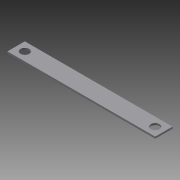
# Autodesk Inventor part: 4barBar
Saved by Autodesk Inventor 2015 SP1 (Build 190203100, 203)
## iProperties
Created: 2015-02-16
Part Number: 4barBar
Material: Generic
Document SubType Name: Modeling
Designer: 55221
Density: 1 g/cm^3
Appearance: Default
Author: 55221
Autodesk Inventor part; units mm, degrees
ref_plane "YZ Plane" through (0, 0, 0) normal (1, 0, 0) x (0, 1, 0)
ref_plane "XZ Plane" through (0, 0, 0) normal (0, 1, 0) x (-1, 0, 0)
ref_plane "XY Plane" through (0, 0, 0) normal (0, 0, 1) x (1, 0, 0)
sketch "Sketch1" plane through (0, 0, 0) normal (0, 1, 0) x (-1, 0, 0)
  line L0 (203.2, 25.4) -> (0, 25.4)
  line L1 (0, 25.4) -> (0, 0)
  line L2 (0, 0) -> (203.2, 0)
  line L3 (203.2, 0) -> (203.2, 25.4)
  constraints: 8 end point, 2 parallel, 1 horizontal, 1 perpendicular
extrude "Extrusion1" add sketch "Sketch1" along normal blind 2.54
sketch "Sketch2" plane through (0, 2.54, 0) normal (0, 1, 0) x (1, 0, 0)
  circle A0 centre (-12.7, -12.7) radius 6.35
  point P0 (0, 0)
  dimension "d2" = 12.7
  constraints: 1 centre point
  measures "d2" diameter of A0
sketch "Sketch3" plane through (-203.2, 0, 0) normal (-1, 0, 0) x (0, 0, 1)
  line L0 (25.4, 0) -> (0, 0) projected
  line L1 (25.4, 0) -> (25.4, 2.54) projected
  line L2 (0, 2.54) -> (25.4, 2.54) projected
  line L3 (0, 0) -> (0, 2.54) projected
extrude "Extrusion2" add sketch "Sketch3" along normal blind 12.7
sketch "Sketch4" plane through (0, 2.54, 0) normal (0, 1, 0) x (1, 0, 0)
  circle A0 centre (-203.2, -12.7) radius 6.35
  point P0 (0, 0)
  dimension "d5" = 12.7
  constraints: 1 centre point
  measures "d5" diameter of A0
extrude "Extrusion3" cut sketch "Sketch4" against normal blind 2.54
extrude "Extrusion4" cut sketch "Sketch2" against normal blind 2.54
body "Solid1"
